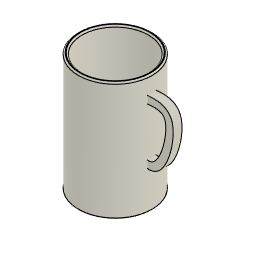
Mug With Handle (Autodesk Fusion 360 design; units mm, degrees)
Autodesk Fusion 360 part; units mm, degrees
note: some values were not read from the file. Set by a fixed rule: which sketch regions a step uses.
sketch "Sketch1" plane through (0, 0, 0) normal (0, 1, 0) x (1, 0, 0)
  line L0 (0, 0) -> (24.5, 0) construction
  line L1 (0, 0) -> (0, -80) construction
  line L2 (25, -0.5) -> (25, -79)
  line L3 (24, -80) -> (23.5, -80)
  line L4 (22.5, 0) -> (22.5, 0)
  line L5 (24.5, 0) -> (22.5, 0)
  arc A0 (22.5, -79) -> (23.5, -80) centre (23.5, -79) ccw
  arc A1 (24, -80) -> (25, -79) centre (24, -79) ccw
  line L6 (0, -4.5) -> (0, -2)
  arc A2 (25, -0.5) -> (24.5, 0) centre (24.5, -0.5) ccw
  line L7 (22.5, -3.6892) -> (22.5, -79)
  line L8 (22.5, -0.5) -> (22.5, -0.5)
  arc A3 (0, -2) -> (22.5, 0) centre (-0.0267, 125.863) ccw
  line L9 (2.5, -4.5) -> (2.5, -4.4755)
  arc A4 (0, -4.5) -> (21.3329, -2.7033) centre (-0.0267, 123.363) ccw
  arc A5 (22.5, -3.6892) -> (21.3329, -2.7033) centre (21.5, -3.6892) ccw
  point P0 (25, -80)
  point P1 (22.5, -80)
  dimension "d2" = 80
  dimension "d3" = 2.5
  dimension "d4" = 1
  dimension "d13" = 1
  constraint coincident L0.start L1.start
  constraint horizontal L0
  constraint perpendicular L0 L1
  constraint perpendicular L0 L2
  constraint perpendicular L2 L3
  constraint coincident L0 L4.start
  constraint coincident P1 L3
  constraint tangent L3 A0
  constraint coincident P0 L2
  constraint coincident P0 L3
  constraint tangent L2 A1
  constraint tangent L3 A1
  constraint equal A0 A1
  constraint coincident L1 L6.end
  constraint coincident L1 L6.start
  constraint coincident L4 A0.start
  constraint tangent L2 A2
  constraint tangent L0 A2
  constraint coincident L4.start L5
  constraint coincident L4.start L8
  constraint parallel L6 L9
  constraint tangent A4 A5
  constraint tangent L7 A5
  measures "d2" distance of L0.start L1.end
  measures "d3" distance of P0 P1
  measures "d4" radius of A0
  measures "d13" radius of A5
revolve "Revolve1" add sketch "Sketch1" angle 360 about axis through (0, 0, 0) along (0, 0, 1) makes body 1
sketch "Sketch2" plane through (0, 0, 0) normal (0, 1, 0) x (1, 0, 0)
  line L0 (-25, -79) -> (25, -79) construction
  spline S0 degree 3 poles (23.6244, -63.5242) (26.5919, -63.9446) (29.2569, -64.0681) (31.4235, -63.8005) (32.8611, -63.6229) (34.0347, -63.2681) (34.8927, -62.6656) (35.6831, -62.1105) (36.2901, -61.3322) (36.7248, -59.9491) (37.1991, -58.4402) (37.3893, -56.1977) (37.1992, -53.4959) (36.8861, -49.0478) (35.5648, -43.4201) (33.7011, -39.0217) (32.5714, -36.3556) (31.2473, -34.1694) (29.9066, -32.7732) (28.7271, -31.5451) (27.5811, -30.92) (26.4128, -30.7428) (25.5599, -30.6135) (24.6555, -30.7137) (23.6244, -31.1024) knots 0 0 0 0 0.174878 0.174878 0.174878 0.290918 0.290918 0.290918 0.397818 0.397818 0.397818 0.514448 0.514448 0.514448 0.706465 0.706465 0.706465 0.822859 0.822859 0.822859 0.925246 0.925246 0.925246 1 1 1 1
  spline S1 degree 3 poles (22.923, -68.4747) (26.1675, -68.9344) (29.189, -69.1145) (32.0364, -68.7627) (33.5555, -68.5751) (35.0763, -68.2364) (36.5968, -67.4599) (36.9912, -67.2585) (37.3836, -67.0261) (37.7662, -66.7573) (38.7165, -66.09) (39.6903, -65.1002) (40.3843, -63.9535) (40.8618, -63.1645) (41.2204, -62.3212) (41.4947, -61.4484) (42.0183, -59.7825) (42.2227, -58.0571) (42.265, -56.1393) (42.2861, -55.1837) (42.26, -54.1852) (42.1868, -53.1449) (41.8982, -49.0439) (40.9337, -44.4541) (39.4934, -40.206) (39.1298, -39.1335) (38.7343, -38.0843) (38.3049, -37.071) (37.2754, -34.6414) (36.0956, -32.4875) (34.6731, -30.6576) (34.3073, -30.1871) (33.9235, -29.7376) (33.5129, -29.3099) (32.3271, -28.0752) (30.9494, -27.0432) (29.3566, -26.401) (28.6483, -26.1154) (27.9052, -25.912) (27.1625, -25.7993) (25.6708, -25.5731) (24.0658, -25.7216) (22.6069, -26.1687) (22.3549, -26.246) (22.1061, -26.3313) (21.8603, -26.424) knots 0 0 0 0 0.174878 0.174878 0.174878 0.267014 0.267014 0.267014 0.290918 0.290918 0.290918 0.354246 0.354246 0.354246 0.397818 0.397818 0.397818 0.475661 0.475661 0.475661 0.514448 0.514448 0.514448 0.667762 0.667762 0.667762 0.706465 0.706465 0.706465 0.799053 0.799053 0.799053 0.822859 0.822859 0.822859 0.89373 0.89373 0.89373 0.925246 0.925246 0.925246 0.98899 0.98899 0.98899 1 1 1 1
  line L1 (23.6244, -31.1024) -> (23.6244, -25.9104)
  line L2 (23.6244, -63.5242) -> (24.1574, -63.4464) construction
  line L3 (23.6244, -68.5701) -> (23.6244, -63.5242) construction
  line L4 (23.6244, -68.5701) -> (23.6244, -63.5242)
  line L5 (-25, -0.5) -> (25, -0.5) construction
  line L6 (25, -0.5) -> (0, -0.5) construction
  point P0 (25, -79)
  point P1 (25, -0.5)
  dimension "d16" = 5
  dimension "d21" = 25
  constraint coincident S1 L1.end
  constraint coincident S1 L3.start
  constraint coincident P1 L5.end
  measures "d21" distance of P1 L6.end
extrude "Extrude1" add sketch "Sketch2" along normal mid plane 6 separate body makes body 2
